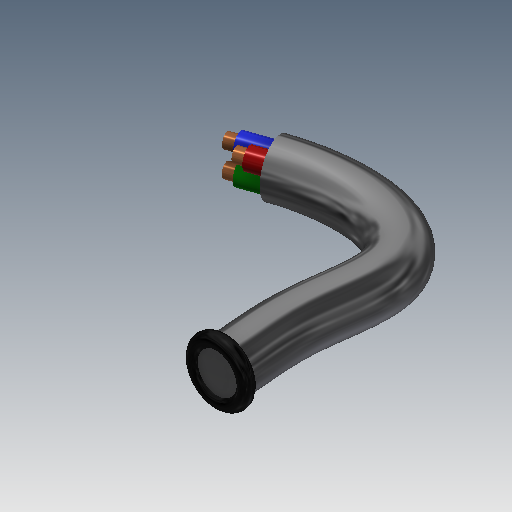
# Autodesk Inventor part: Part1
Saved by Autodesk Inventor 2019.1 (Build 231200000, 200)
## iProperties
Created: 2007-02-07
Part Number: Part1
Document SubType Name: Modeling
Designer: Stephen Hooper
Density: 1 g/cm^3
Material: Generic
Mass: 19.0059 g
Surface Area: 58.8285 cm^2
Volume: 19.0059 cm^3
Appearance: Rubber - Black - Version 1.1
Author: Stephen Hooper
Autodesk Inventor part; units mm, degrees
ref_plane "XY Plane" through (0, 0, 0) normal (0, 0, 1) x (1, 0, 0)
sketch "Sketch1" plane through (0, 0, 0) normal (0, 0, 1) x (1, 0, 0)
  circle A0 centre (-17.5, 48) radius 7.5 projected
  point P0 (0, 0)
ref_plane "Work Plane1" through (-17.5, 48, 0) normal (1, 0, 0) x (0, 1, 0)
ref_plane "Work Plane2" through (-17.5, 48, 0) normal (0, 1, 0) x (-1, 0, 0)
sketch "Sketch2" plane through (-17.5, 48, 0) normal (0, 1, 0) x (-1, 0, 0)
  spline S0 degree 4 poles (0, 0) (0, -12.2101) (7.249, -30.6467) (-16.4407, -58.3105) (21.0008, -68.9176) (43.9349, -61.0095) knots 0 0 0 0 0 0.479571 1 1 1 1 1
  line L0 (0, 9.4013) -> (0, -9.4013) construction
  arc A0 (0.4883, 7.4568) -> (0.4883, -7.4568) centre (57.1813, 0) ccw construction
  line L1 (-7.5, 0) -> (7.5, 0) construction
  line L2 (31.8572, -65.1742) -> (56.0127, -56.8449) construction
  arc A1 (34.1338, -63.5881) -> (53.2424, -56.9991) centre (21.828, 3.1026) ccw construction
  point P0 (-48, 0)
  point P1 (0.8767, -27.7866)
  point P2 (0.5269, -52.3931)
  constraints: 6 end point, 4 midpoint, 2 centre point, 2 point on circle, 1 perpendicular, 1 vertical, 7 other
sweep "Sweep1" add profiles "Sketch1" path "Sketch2"
sketch "Sketch3" plane through (-61.4349, 48, -61.0095) normal (-0.9453761, 0, 0.3259817) x (0.3259817, 0, 0.9453761)
  circle A0 centre (0, 0) radius 7.5 projected
  circle A1 centre (0, 0) radius 6.5
  circle A2 centre (2.444, 2.4821) radius 3.0167
  circle A3 centre (-3.3715, 0.8755) radius 3.0167
  circle A4 centre (0.9275, -3.3576) radius 3.0167
  point P0 (-7.5, 0)
  point P1 (77.7036, -48)
  dimension "d1" = 1
  constraints: 6 tangent, 4 centre point, 2 equal radius, 1 horizontal alignment
extrude "Extrusion1" add sketch "Sketch3" along normal blind 5 contours A2
extrude "Extrusion2" add sketch "Sketch3" along normal blind 10 contours A3
extrude "Extrusion3" add sketch "Sketch3" along normal blind 8 contours A4
sketch "Sketch4" plane through (-71.9877, 48.8755, -60.9371) normal (-0.9453761, 0, 0.3259817) x (0.3259817, 0, 0.9453761)
  circle A0 centre (0, 0) radius 3.0167 projected
  circle A1 centre (0, 0) radius 2.0167
  point P0 (81.0751, -48.8755)
  dimension "d8" = 1
  constraints: 1 centre point
  measures "d8" radial gap between concentric circles of A0 A1
sketch "Sketch5" plane through (-66.1618, 48, -59.3796) normal (-0.9453761, 0, 0.3259817) x (0.3259817, 0, 0.9453761)
  arc A0 (1.6858, -0.4378) -> (-0.4638, 1.6788) centre (2.444, 2.4821) ccw projected
  arc A1 (-0.4638, 1.6788) -> (1.6858, -0.4378) centre (2.444, 2.4821) ccw projected
  arc A2 (1.9371, 0.5301) -> (0.5001, 1.9451) centre (2.444, 2.4821) ccw
  arc A3 (0.5001, 1.9451) -> (1.9371, 0.5301) centre (2.444, 2.4821) ccw
  point P0 (77.7036, -48)
  dimension "d9" = 1
  constraints: 4 point on circle, 2 centre point, 1 other
  measures "d9" radial gap between concentric circles of A0 A2
sketch "Sketch6" plane through (-68.6956, 44.6424, -57.5248) normal (-0.9453761, 0, 0.3259817) x (0.3259817, 0, 0.9453761)
  circle A0 centre (0, 0) radius 3.0167 projected
  circle A1 centre (0, 0) radius 2.0167
  point P0 (-2.1495, 2.1165)
  point P1 (76.7761, -44.6424)
  dimension "d10" = 1
  constraints: 1 centre point, 1 other
extrude "Extrusion4" add sketch "Sketch4" along normal blind 3 contours A1
extrude "Extrusion5" add sketch "Sketch6" along normal blind 3 contours A1
extrude "Extrusion6" add sketch "Sketch5" along normal blind 3 contours A3 A2
sketch "Sketch7" plane through (-17.5, 48, 0) normal (1, 0, 0) x (0, 1, 0)
  line L0 (7.5, -1) -> (-7.5, -1) projected
  circle A0 centre (-7.5, -1) radius 2
  line L1 (0, -1.369) -> (0, -7.6638)
  point P0 (-48, 0)
  dimension "d17" = 4
  constraints: 2 end point, 1 centre point, 1 coincident, 1 perpendicular
  measures "d17" diameter of A0
revolve "Revolution1" add sketch "Sketch7" angle 360 about axis through (-17.5, 48, -1.369) along (0, 0, -1)
body "Solid1"
